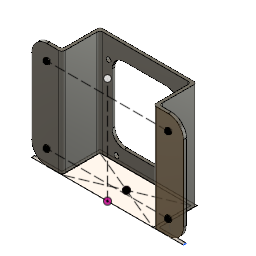
radarbeugel (Autodesk Fusion 360 design; units mm, degrees)
Autodesk Fusion 360 part; units mm, degrees
sketch "Sketch1" plane through (0, 0, 0) normal (0, 1, 0) x (1, 0, 0)
  line L0 (30, 12.5) -> (-30, 12.5)
  line L1 (-30, 12.5) -> (-30, -12.5)
  line L2 (-30, -12.5) -> (30, -12.5)
  line L3 (30, -12.5) -> (30, 12.5)
  line L4 (30, 12.5) -> (-30, -12.5) construction
  line L5 (-30, 12.5) -> (30, -12.5) construction
  line L6 (-30, -12.5) -> (-50, -12.5)
  line L7 (-50, -12.5) -> (-50, -10.5)
  line L8 (-50, -10.5) -> (-32, -10.5)
  line L9 (-32, -10.5) -> (-32, 14.5)
  line L10 (-32, 14.5) -> (32, 14.5)
  line L11 (32, 14.5) -> (32, -10.5)
  line L12 (32, -10.5) -> (50, -10.5)
  line L13 (50, -10.5) -> (50, -12.5)
  line L14 (50, -12.5) -> (30, -12.5)
  dimension "d1" = 60
  dimension "d2" = 25
  dimension "d3" = 20
  dimension "d4" = 2
  dimension "d6" = 18
  dimension "d7" = 25
  dimension "d8" = 64
  dimension "d9" = 25
  dimension "d10" = 2
  constraint perpendicular L0 L1
  constraint parallel L0 L2
  constraint parallel L1 L3
  constraint horizontal L0
  constraint coincident L4 origin
  constraint coincident L5 origin
  constraint perpendicular L1 L6
  constraint perpendicular L6 L7
  constraint perpendicular L1 L8
  constraint perpendicular L8 L9
  constraint perpendicular L9 L10
  constraint perpendicular L0 L11
  constraint perpendicular L11 L12
  constraint perpendicular L12 L13
  measures "d1" distance of L1.end L2.end
  measures "d2" distance of L0.end L1.end
  measures "d3" distance of L1.end L6.end
  measures "d4" distance of L6.end L7.end
  measures "d6" distance of L7.end L8.end
  measures "d7" distance of L8.end L9.end
  measures "d8" distance of L9.end L10.end
  measures "d9" distance of L10.end L11.end
  measures "d10" distance of L12.end L13.end
extrude "Extrude1" add sketch "Sketch1" along normal blind 70 contours L0 L1 L3 L6 L7 L8 L9 L10 L11 L12 L13 L14
sketch "Sketch2" plane through (0, 0, -14.5) normal (0, 0, -1) x (-1, 0, 0)
  line L0 (-32, 0) -> (32, 0)
  line L1 (32, 0) -> (32, 70)
  line L2 (32, 70) -> (-32, 70)
  line L3 (-32, 70) -> (-32, 0)
  line L4 (0, 70) -> (0, 0) construction
  line L5 (0, 70) -> (0, 54.76) construction
  line L6 (0, 54.76) -> (0, 56.03)
  line L7 (0, 56.03) -> (24.257, 56.03) construction
  line L8 (0, 54.76) -> (-24.13, 54.76) construction
  circle A0 centre (-24.13, 54.76) radius 1.6
  circle A1 centre (24.257, 56.03) radius 1.6
  line L9 (-24.13, 54.76) -> (-24.13, 3.96) construction
  line L10 (-24.13, 3.96) -> (-8.89, 3.96) construction
  circle A2 centre (-8.89, 3.96) radius 1.6
  line L11 (-8.89, 3.96) -> (19.05, 3.96) construction
  circle A3 centre (19.05, 3.96) radius 1.6
  circle A4 centre (-24.13, 54.76) radius 3.2
  circle A5 centre (24.257, 56.03) radius 3.2
  line L12 (-14, 10) -> (14, 10)
  line L13 (22, 18) -> (22, 52)
  line L14 (14, 60) -> (-14, 60)
  line L15 (-22, 52) -> (-22, 18)
  arc A6 (-14, 60) -> (-22, 52) centre (-14, 52) ccw
  arc A7 (22, 52) -> (14, 60) centre (14, 52) ccw
  arc A8 (14, 10) -> (22, 18) centre (14, 18) ccw
  arc A9 (-22, 18) -> (-14, 10) centre (-14, 18) ccw
  dimension "d13" = 15.24
  dimension "d16" = 1.27
  dimension "d19" = 24.257
  dimension "d20" = 24.13
  dimension "d21" = 3.2
  dimension "d22" = 3.2
  dimension "d23" = 50.8
  dimension "d24" = 15.24
  dimension "d25" = 3.2
  dimension "d26" = 27.94
  dimension "d27" = 3.2
  dimension "d41" = 6.4
  dimension "d42" = 6.4
  dimension "d44" = 8
  dimension "d45" = 8
  dimension "d46" = 8
  dimension "d47" = 8
  constraint midpoint L2 L4.start
  constraint coincident L4.end origin
  constraint perpendicular L2 L5
  constraint perpendicular L6 L7
  constraint perpendicular L6 L8
  constraint coincident L8.end A0.centre
  constraint coincident L7.end A1.centre
  constraint perpendicular L8 L9
  constraint perpendicular L9 L10
  constraint coincident L10.end A2.centre
  constraint perpendicular L4 L11
  constraint coincident L11.end A3.centre
  constraint concentric A1 A5
  constraint parallel L0 L12
  constraint parallel L1 L13
  constraint parallel L2 L14
  constraint parallel L3 L15
  constraint tangent L14 A6
  constraint tangent L15 A6
  constraint tangent L13 A7
  constraint tangent L14 A7
  constraint tangent L12 A8
  constraint tangent L13 A8
  constraint tangent L12 A9
  constraint tangent L15 A9
  measures "d13" distance of L4.start L5.end
  measures "d16" distance of L5.end L6.end
  measures "d19" distance of L6.end L7.end
  measures "d20" distance of L5.end L8.end
  measures "d21" diameter of A0
  measures "d22" diameter of A1
  measures "d23" distance of L8.end L9.end
  measures "d24" distance of L9.end L10.end
  measures "d25" diameter of A2
  measures "d26" distance of L10.end L11.end
  measures "d27" diameter of A3
  measures "d41" diameter of A4
  measures "d42" diameter of A5
  measures "d44" radius of A6
  measures "d45" radius of A7
  measures "d46" radius of A8
  measures "d47" radius of A9
extrude "Extrude4" cut sketch "Sketch2" against normal blind 2 contours A4 A5 L12 L13 L14 L15 A6 A7 A8 A9
extrude "Extrude2" cut sketch "Sketch2" against normal blind 2 contours A0 | A1 | A2 | A3
fillet "Fillet1" radius 10 4 edges at (-50, 70, 11.5) (50, 70, 11.5) (50, 0, 11.5) (-50, 0, 11.5)
fillet "Fillet2" radius 2 8 edges at (-30, 35, 12.5) (-30, 35, -12.5) (30, 35, -12.5) (30, 35, 12.5) (32, 35, 10.5) (32, 35, -14.5) (-32, 35, -14.5) (-32, 35, 10.5)
sketch "Sketch3" plane through (0, 0, 12.5) normal (0, 0, 1) x (1, 0, 0)
  line L0 (32, 70) -> (32, 0)
  line L1 (32, 0) -> (40, 0)
  arc A0 (40, 0) -> (50, 10) centre (40, 10) ccw
  line L2 (50, 10) -> (50, 60)
  arc A1 (50, 60) -> (40, 70) centre (40, 60) ccw
  line L3 (40, 70) -> (32, 70)
  circle A2 centre (40, 60) radius 2
  circle A3 centre (40, 10) radius 2
  line L4 (0, 0) -> (0, 70) construction
  line L5 (40, 60) -> (-40, 60) construction
  line L6 (40, 10) -> (-40, 10) construction
  circle A4 centre (-40, 60) radius 2
  circle A5 centre (-40, 10) radius 2
  dimension "d32" = 4
  dimension "d33" = 4
  dimension "d34" = 80
  dimension "d35" = 80
  dimension "d36" = 4
  dimension "d37" = 4
  constraint concentric A1 A2
  constraint concentric A0 A3
  constraint coincident L4.start origin
  constraint vertical L4
  constraint coincident A1.centre A2.centre
  constraint horizontal L5
  constraint coincident A0.centre A3.centre
  constraint horizontal L6
  constraint coincident L5.end A4.centre
  constraint coincident L6.end A5.centre
  measures "d32" diameter of A2
  measures "d33" diameter of A3
  measures "d34" distance of A1.centre L5.end
  measures "d35" distance of A0.centre L6.end
  measures "d36" diameter of A4
  measures "d37" diameter of A5
extrude "Extrude3" cut sketch "Sketch3" against normal blind 2 contours A2 | A3 | A4 | A5
equation "d4 = width"
equation "width = 2 mm"
equation "d6 = 20 mm - width"
equation "d8 = 60 mm + 2 * width"
equation "d10 = width"
equation "d28 = -width"
equation "d38 = -width"
equation "d48 = -width"
